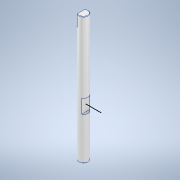
# Autodesk Inventor part: shaft
Saved by Autodesk Inventor 2022 (Build 260153000, 153)
## iProperties
Created: 2022-04-20
Part Number: shaft
Material: アルミニウム 6061
Document SubType Name: Modeling
Designer: Yazawa
Density: 2.7 g/cm^3
Appearance: アルミニウム - フラット
Author: Yazawa
Autodesk Inventor part; units mm, degrees
ref_plane "YZ Plane" through (0, 0, 0) normal (1, 0, 0) x (0, 1, 0)
ref_plane "XZ Plane" through (0, 0, 0) normal (0, 1, 0) x (-1, 0, 0)
ref_plane "XY Plane" through (0, 0, 0) normal (0, 0, 1) x (1, 0, 0)
sketch "スケッチ1" plane through (0, 0, 0) normal (0, 1, 0) x (-1, 0, 0)
  circle A0 centre (0, 0) radius 2
  dimension "d0" = 4
  constraints: 1 centre point, 1 coincident
  measures "d0" diameter of A0
extrude "押し出し1" add sketch "スケッチ1" along normal blind 55
sketch "スケッチ2" plane through (0, 55, 0) normal (0, 1, 0) x (1, 0, 0)
  circle A0 centre (0, 0) radius 2 projected
  line L0 (-1, -1.7321) -> (-1, 1.7321)
  dimension "d3" = 1
  constraints: 2 end point, 2 point on circle, 1 vertical
  measures "d3" distance from line of L0 point (0, 0)
extrude "押し出し2" cut sketch "スケッチ2" against normal blind 5 contours L0 A0 picked at (-1.1242, -0.4849)
chamfer "面取り1" distance 0.2 angle 45 2 edges at (2, 55, 0) (2, 0, 0)
sketch "スケッチ3" plane through (0, 0, 0) normal (0, 0, 1) x (1, 0, 0)
  line L0 (1, 18.4) -> (2, 18.4)
  line L1 (2, 18.4) -> (2, 21.4)
  line L2 (2, 21.4) -> (1, 21.4)
  line L3 (1, 21.4) -> (1, 18.4)
  line L4 (1.8, 0) -> (-1.8, 0) projected
  line L5 (1, 24.4) -> (2, 24.4)
  line L6 (2, 24.4) -> (2, 21.4)
  line L7 (1, 21.4) -> (1, 24.4)
  line L8 (2, 0.2) -> (2, 54.8) projected
  point P0 (0, 0)
  dimension "d9" = 1
  dimension "d10" = 3
  dimension "d11" = 21.4
  constraints: 14 end point, 2 parallel, 2 symmetric about line, 1 collinear, 1 horizontal, 1 perpendicular
  measures "d9" distance of L2.end L1.end
  measures "d10" distance of L1.end L0.end
  measures "d11" distance between parallel lines of L4 L2
extrude "押し出し3" cut sketch "スケッチ3" along normal mid plane 55
ref_plane "作業平面1" through (0, 21.4, 0) normal (0, 1, 0) x (1, 0, 0)
sketch "スケッチ5" plane through (0, 21.4, 0) normal (0, 1, 0) x (1, 0, 0)
  line L0 (0, 0) -> (7.6217, 0)
  constraints: 2 end point, 1 horizontal
